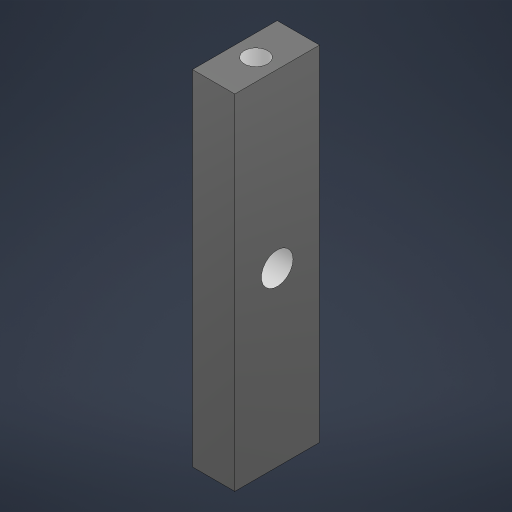
# Autodesk Inventor part: BallSensor
Saved by Autodesk Inventor 2024.2 (Build 282272000, 272)
## iProperties
Created: 2023-12-28
Part Number: BallSensor
Material: 一般
Document SubType Name: Modeling
Designer: Hanaoka
Density: 1 g/cm^3
Appearance: 既定
Author: Hanaoka
Autodesk Inventor part; units mm, degrees
ref_plane "YZ Plane" through (0, 0, 0) normal (1, 0, 0) x (0, 1, 0)
ref_plane "XZ Plane" through (0, 0, 0) normal (0, 1, 0) x (-1, 0, 0)
ref_plane "XY Plane" through (0, 0, 0) normal (0, 0, 1) x (1, 0, 0)
sketch "スケッチ1" plane through (0, 0, 0) normal (0, 1, 0) x (-1, 0, 0)
  line L0 (-2, 4) -> (2, 4)
  line L1 (2, 4) -> (2, -4)
  line L2 (2, -4) -> (-2, -4)
  line L3 (-2, -4) -> (-2, 4)
  line L4 (-2, 4) -> (2, -4) construction
  line L5 (2, 4) -> (-2, -4) construction
  circle A0 centre (0, 0) radius 1
  dimension "d0" = 8
  dimension "d1" = 4
  dimension "d2" = 2
  constraints: 12 end point, 2 midpoint, 2 parallel, 1 centre point, 1 coincident, 1 horizontal, 1 perpendicular
  measures "d0" distance of L0.end L1.end
  measures "d1" distance of L1.end L2.end
  measures "d2" diameter of A0
extrude "押し出し1" add sketch "スケッチ1" along normal blind 32.5 contours L0 L1 L2 L3 | A0
sketch "スケッチ2" plane through (0, 0, 0) normal (0, -1, 0) x (1, 0, 0)
  circle A0 centre (0, 0) radius 0.8
  dimension "d5" = 1.6
  constraints: 1 centre point, 1 coincident
  measures "d5" diameter of A0
extrude "押し出し2" cut sketch "スケッチ2" against normal blind 6
sketch "スケッチ3" plane through (2, 0, 4) normal (1, 0, 0) x (0, 0, -1)
  circle A0 centre (4, 24.25) radius 1.5 construction
  circle A1 centre (4, 8.25) radius 1.5 construction
  line L0 (8, 32.5) -> (0, 32.5) projected
  line L1 (4, 32.5) -> (4, 0)
  line L2 (4, 0) -> (3.3318, 0)
  line L3 (4, 32.5) -> (4, 24.25) construction
  line L4 (4, 24.25) -> (4, 8.25) construction
  line L5 (4, 8.25) -> (4, 0) construction
  line L6 (0, 0) -> (8, 0) projected
  line L7 (0, 32.5) -> (8, 32.5) projected
  circle A2 centre (4, 16.25) radius 1.5
  dimension "d8" = 3
  dimension "d9" = 16
  dimension "d15" = 3
  constraints: 10 end point, 4 midpoint, 3 centre point, 3 point on line, 2 vertical, 1 collinear, 1 equal radius
  measures "d8" diameter of A1
  measures "d9" distance of L4.end L3.end
  measures "d15" diameter of A2
extrude "押し出し3" cut sketch "スケッチ3" against normal up to surface (4 mm away)
sketch "スケッチ4" plane through (0, 32.5, 0) normal (0, 1, 0) x (1, 0, 0)
  circle A0 centre (0, 0) radius 1.1
  dimension "d12" = 2.2
  constraints: 1 centre point, 1 coincident
  measures "d12" diameter of A0
extrude "押し出し4" cut sketch "スケッチ4" against normal blind 6
